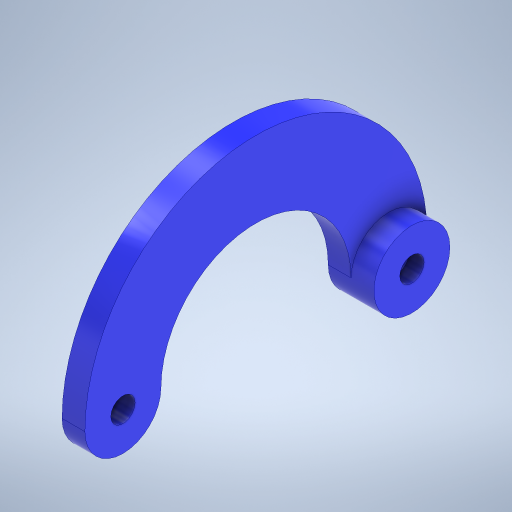
# Autodesk Inventor part: endeff_3dp3
Saved by Autodesk Inventor 2024 (Build 280153000, 153)
## iProperties
Created: 2024-12-14
Part Number: endeff_3dp3
Material: ABS プラスチック
Document SubType Name: Modeling
Designer: hirek
Density: 1.06 g/cm^3
Appearance: 青 - 壁塗料 - 光沢
Author: hirek
Autodesk Inventor part; units mm, degrees
ref_plane "YZ Plane" through (0, 0, 0) normal (1, 0, 0) x (0, 1, 0)
ref_plane "XZ Plane" through (0, 0, 0) normal (0, 1, 0) x (-1, 0, 0)
ref_plane "XY Plane" through (0, 0, 0) normal (0, 0, 1) x (1, 0, 0)
sketch "スケッチ1" plane through (0, 0, 0) normal (1, 0, 0) x (0, 1, 0)
  circle A0 centre (0, 0) radius 5
  circle A1 centre (0, -35) radius 5
  line L0 (0, 0) -> (0, -35)
  circle A2 centre (0, -17.5) radius 12.5
  circle A3 centre (0, -17.5) radius 22.5
  point P0 (0, 5)
  point P1 (0, -5)
  point P2 (0, -30)
  point P3 (0, -40)
  dimension "d0" = 10
  dimension "d1" = 10
  dimension "d2" = 35
  constraints: 4 centre point, 2 coincident, 2 end point, 2 tangent, 1 midpoint, 1 vertical
  measures "d0" diameter of A0
  measures "d1" diameter of A1
  measures "d2" distance of L0.end point (0, 0)
extrude "押し出し1" add sketch "スケッチ1" along normal blind 3 contours A0 | A0 A3 A1 A2 | A1 picked at (8.8989, -32.0838)
sketch "スケッチ2" plane through (3, 0, 0) normal (1, 0, 0) x (0, 0, -1)
  arc A0 (30, 0) -> (40, 0) centre (35, 0) ccw projected
  circle A1 centre (35, 0) radius 5
  point P0 (0, 0)
  point P1 (40, 0)
  point P2 (30, 0)
  dimension "d5" = 10
  constraints: 1 centre point, 1 coincident
  measures "d5" diameter of A1
extrude "押し出し2" add sketch "スケッチ2" along normal blind 3
sketch "スケッチ3" plane through (0, 0, 0) normal (-1, 0, 0) x (0, 0, 1)
  arc A0 (-40, 0) -> (-30, 0) centre (-35, 0) ccw projected
  arc A1 (-5, 0) -> (5, 0) centre (0, 0) ccw projected
  constraints: 2 coincident
hole "穴1" at (0, 0, -35) at (0, 0, 0) direction (1, 0, 0) diameter 3.2 end through all
sketch "スケッチ4" plane through (0, 0, 0) normal (-1, 0, 0) x (0, 0, 1)
  circle A0 centre (-35, 0) radius 1.6 projected
  circle A1 centre (-35, 0) radius 3.5
  point P0 (0, 0)
  dimension "d15" = 7
  constraints: 1 centre point, 1 coincident
  measures "d15" diameter of A1
extrude "押し出し3" cut sketch "スケッチ4" against normal blind 4
